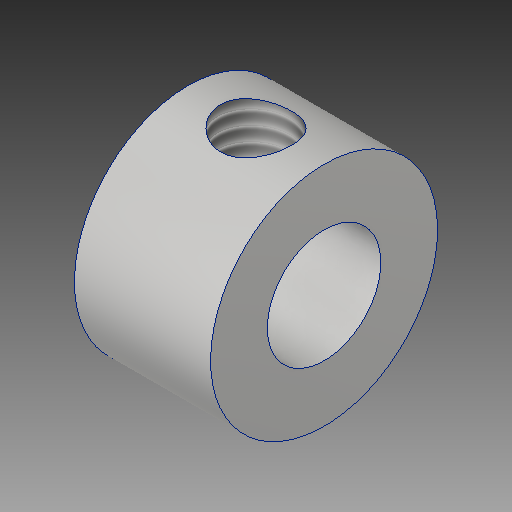
# Autodesk Inventor part: Collar
Saved by Autodesk Inventor 2019 (Build 230136000, 136)
## iProperties
Created: 2018-04-18
Part Number: Collar
Material: Aluminum 6061
Document SubType Name: Modeling
Designer: User
Density: 2.7 g/cm^3
Appearance: Aluminum - Flat
Mass: 1.73436 g
Surface Area: 6.39619 cm^2
Volume: 0.642356 cm^3
Author: User
Autodesk Inventor part; units mm, degrees
ref_plane "YZ Plane" through (0, 0, 0) normal (1, 0, 0) x (0, 1, 0)
ref_plane "XZ Plane" through (0, 0, 0) normal (0, 1, 0) x (-1, 0, 0)
sketch "Sketch2" plane through (0, 0, 0) normal (0, 0, 1) x (1, 0, 0)
  line L0 (0, 0) -> (7.62, 0)
  line L1 (-0.4445, 6.35) -> (7.1755, 6.35)
  line L2 (7.1755, 6.35) -> (7.1755, 3.175)
  line L3 (7.1755, 3.175) -> (-0.4445, 3.175)
  line L4 (-0.4445, 3.175) -> (-0.4445, 6.35)
  point P0 (3.3655, 6.35)
  dimension "d8" = 7.62
  dimension "d9" = 3.175
  dimension "d10" = 7.62
  dimension "d11" = 3.175
  constraints: 10 end point, 2 horizontal, 2 parallel, 1 midpoint, 1 perpendicular
  measures "d8" distance of L0.start L0.end
  measures "d9" distance of L1.end L2.end
  measures "d10" distance of L1.start L1.end
  measures "d11" distance between parallel lines of L0 L3
revolve "Revolution1" add sketch "Sketch2" angle 360 about axis through (0, 0, 0) along (1, 0, 0)
ref_plane "Work Plane1" through (3.3655, 6.35, 0) normal (0, 1, 0) x (-1, 0, 0)
sketch "Sketch3" plane through (3.3655, 6.35, 0) normal (0, 1, 0) x (-1, 0, 0)
  point P0 (3.3655, 0)
  point P1 (0, 0)
hole "Hole1" at (3.3655, 6.35, 0) direction (0, -1, 0) diameter 3.9624 depth 3.175 tip angle 118 thread size "10-32 UNF" class "2B" standard "ANSI Unified Screw Threads"
equation "\"d10\" = d8"
body "Solid2"
